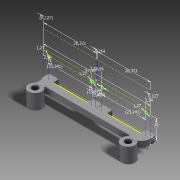
# Autodesk Inventor part: HDMIPluginModuleHolder02
Saved by Autodesk Inventor 2015 (Build 190159000, 159)
## iProperties
Created: 2015-10-14
Part Number: HDMIPluginModuleHolder02
Material: Generic
Document SubType Name: Modeling
Designer: -
Density: 1 g/cm^3
Appearance: Default
Author: -
Autodesk Inventor part; units mm, degrees
ref_plane "YZ Plane" through (0, 0, 0) normal (1, 0, 0) x (0, 1, 0)
ref_plane "XZ Plane" through (0, 0, 0) normal (0, 1, 0) x (-1, 0, 0)
ref_plane "XY Plane" through (0, 0, 0) normal (0, 0, 1) x (1, 0, 0)
sketch "Sketch1" plane through (0, 0, 0) normal (0, 1, 0) x (-1, 0, 0)
  circle A0 centre (0, 0) radius 1.65
  line L0 (0, 0) -> (22.8671, 0) construction
  circle A1 centre (-49.53, 0) radius 1.65
  circle A2 centre (-49.53, 0) radius 3.5
  line L1 (-24.765, 0) -> (-24.765, 33.4897) construction
  line L2 (0, 0) -> (0, -6.322) construction
  line L3 (-49.53, 0) -> (-44.53, 0) construction
  circle A3 centre (0, 0) radius 3.5
  dimension "d0" = 3.3
  dimension "d2" = 49.53
  dimension "d3" = 3.3
  dimension "d4" = 7
  dimension "d11" = 7
  constraints: 8 end point, 4 centre point, 3 coincident, 2 horizontal, 2 vertical, 1 point on line
  measures "d0" diameter of A0
  measures "d2" distance of L0.start A1.centre
  measures "d3" diameter of A1
  measures "d4" diameter of A2
  measures "d11" diameter of A3
extrude "Extrusion1" add sketch "Sketch1" along normal blind 3
sketch "Sketch2" plane through (49.53, 0, 0) normal (0, -1, 0) x (1, 0, 0)
  line L0 (2, -2.2) -> (2, -5.2)
  line L1 (0, -7.2) -> (-49.53, -7.2)
  line L2 (-51.53, -5.2) -> (-51.53, -2.2)
  line L3 (-47.53, -2.2) -> (-47.53, -2.2)
  line L4 (-46.53, -3.2) -> (-3, -3.2)
  line L5 (-2, -2.2) -> (-2, -2.2)
  line L6 (0, 0) -> (0, -7.7115) construction
  line L7 (2, -2.2) -> (-2, -2.2)
  line L8 (-49.53, 0) -> (-49.53, -7.2415) construction
  line L9 (-47.53, -2.2) -> (-51.53, -2.2)
  arc A0 (-47.53, -2.2) -> (-46.53, -3.2) centre (-46.53, -2.2) ccw
  arc A1 (-3, -3.2) -> (-2, -2.2) centre (-3, -2.2) ccw
  arc A2 (-51.53, -5.2) -> (-49.53, -7.2) centre (-49.53, -5.2) ccw
  arc A3 (0, -7.2) -> (2, -5.2) centre (0, -5.2) ccw
  point P0 (2, -7.2)
  point P1 (0, -2.2)
  point P2 (-49.53, -2.2)
  dimension "d14" = 5
  dimension "d15" = 2.2
  dimension "d16" = 4
  dimension "d17" = 4
  dimension "d18" = 2.2
  dimension "d19" = 1
  dimension "d20" = 2
  constraints: 20 end point, 8 point on circle, 8 tangent, 4 centre point, 4 perpendicular, 4 point on line, 3 vertical, 2 equal radius, 2 horizontal, 2 midpoint, 2 other
  measures "d14" distance of L0.start point (2, -7.2)
  measures "d15" distance from line of L6.start L7
  measures "d16" distance between parallel lines of L0 L5
  measures "d17" distance between parallel lines of L4 L1
  measures "d18" distance from line of L8.start L9
  measures "d19" radius of A0
  measures "d20" radius of A2
extrude "Extrusion2" add sketch "Sketch2" against normal blind 3.072
sketch "Sketch3" plane through (49.53, 0, -7.2) normal (0, 0, -1) x (-1, 0, 0)
  arc A0 (20.5268, 0.572) -> (21.6698, 0.572) centre (21.0983, 0.572) ccw
  line L0 (0, 0) -> (49.53, 0) construction
  line L1 (0, 3.072) -> (49.53, 3.072) projected
  line L2 (-2, 0) -> (-2, 3.072) projected
  line L3 (21.6698, 0.572) -> (21.6698, 1.207)
  line L4 (21.6698, 1.207) -> (23.6698, 1.207)
  line L5 (23.6698, 1.207) -> (23.6698, 3.072)
  line L6 (20.5268, 0.572) -> (20.5268, 1.207)
  line L7 (20.5268, 1.207) -> (18.5268, 1.207)
  line L8 (18.5268, 1.207) -> (18.5268, 3.072)
  line L9 (21.0983, 0.572) -> (22.2732, 0.572) construction
  line L10 (23.6698, 3.072) -> (18.5268, 3.072)
  point P0 (49.53, 0)
  point P1 (46.53, 3.072)
  point P2 (3, 3.072)
  dimension "d23" = 1.143
  dimension "d26" = 23.0983
  dimension "d27" = 2
  dimension "d28" = 2
  dimension "d29" = 0.635
  dimension "d30" = 0.635
  dimension "d31" = 2.5
  constraints: 16 end point, 3 perpendicular, 2 collinear, 2 horizontal, 2 point on circle, 2 point on line, 2 vertical, 1 centre point, 1 coincident, 1 tangent
  measures "d23" diameter of A0
  measures "d26" distance from line of A0.centre L2
  measures "d27" distance of L3.end L4.end
  measures "d28" distance of L6.end L7.end
  measures "d29" distance of L6.start L6.end
  measures "d30" distance of L3.start L3.end
  measures "d31" distance from line of L9.start L10
extrude "Extrusion3" add sketch "Sketch3" along normal blind 3
pattern_linear "Rectangular Pattern1" count 2 spacing 23.241 along (1, 0, 0) of "Extrusion3"
sketch "Sketch4" plane through (49.1012, 3.072, -7.2) normal (0, 1, 0) x (1, 0, 0)
  arc A0 (0, -5.143) -> (5.143, 0) centre (0, 0) ccw
  line L0 (5.143, 0) -> (0, 0)
  line L1 (0, 0) -> (0, -5.143)
  point P0 (-49.1012, -7.2)
  constraints: 4 end point, 2 point on circle, 1 centre point, 1 horizontal, 1 perpendicular
extrude "Extrusion4" add sketch "Sketch4" against normal blind 3.072
pattern_linear "Rectangular Pattern2" count 2 spacing 5.334 along (-1, 0, 0) of "Extrusion3"
pattern_linear "Rectangular Pattern3" count 2 spacing 28.575 along (-1, 0, 0) of "Extrusion3"
sketch "Sketch6" plane through (-2.7148, 3.072, -7.2) normal (0, 1, 0) x (1, 0, 0)
  arc A0 (0, 0) -> (3.143, -3.143) centre (3.143, 0) ccw
  line L0 (3.143, -3.143) -> (3.143, 0)
  line L1 (3.143, 0) -> (0, 0)
  point P0 (2.7148, -7.2)
  constraints: 4 end point, 2 point on circle, 1 centre point, 1 perpendicular, 1 vertical
extrude "Extrusion5" add sketch "Sketch6" against normal blind 3.072
sketch "Sketch7" plane through (54.2442, 3.072, -10.2) normal (0, 0, -1) x (-1, 0, 0)
  line L0 (3.143, -2.5) -> (3.143, -1.865) construction
  line L1 (3.143, -1.865) -> (5.143, -1.865) construction
  line L2 (5.143, -1.865) -> (5.143, 0) construction
  line L3 (5.143, 0) -> (0, 0) construction
  line L4 (0, 0) -> (0, -1.865) construction
  line L5 (0, -1.865) -> (2, -1.865) construction
  line L6 (2, -1.865) -> (2, -2.5) construction
  arc A0 (2, -2.5) -> (3.143, -2.5) centre (2.5715, -2.5) ccw construction
  line L7 (0, -1.865) -> (0, 0)
  line L8 (0, 0) -> (5.143, 0)
  line L9 (5.143, 0) -> (5.143, -1.865)
  arc A1 (0, -1.865) -> (5.143, -1.865) centre (2.5715, -1.865) ccw
  line L10 (5.143, -1.865) -> (0, -1.865) construction
  line L11 (5.143, -1.865) -> (5.143, 0) construction
  point P0 (54.2442, -3.072)
  constraints: 8 end point, 3 perpendicular, 2 point on circle, 1 centre point, 1 coincident, 1 midpoint, 1 vertical
extrude "Extrusion6" add sketch "Sketch7" against normal blind 1
pattern_linear "Rectangular Pattern4" count 2 spacing 23.241 along (-1, 0, 0) of "Extrusion6"
pattern_linear "Rectangular Pattern5" count 2 spacing 28.575 along (-1, 0, 0) of "Extrusion6"
pattern_linear "Rectangular Pattern6" count 2 spacing 51.816 along (-1, 0, 0) of "Extrusion6"
sketch "Sketch8" plane through (49.53, 0, -7.2) normal (0, 0, -1) x (-1, 0, 0)
  line L0 (-4.8097, 14.0243) -> (52.3403, 14.0243) construction
  line L1 (52.3403, 14.0243) -> (52.3403, 4.0243) construction
  line L2 (52.3403, 4.0243) -> (-4.8097, 4.0243) construction
  line L3 (-4.8097, 4.0243) -> (-4.8097, 14.0243) construction
  line L4 (-4.6827, 25.3025) -> (23.6383, 25.3025) construction
  line L5 (23.6383, 25.3025) -> (23.6383, 16.2547) construction
  line L6 (23.6383, 16.2547) -> (-4.6827, 16.2547) construction
  line L7 (-4.6827, 16.2547) -> (-4.6827, 25.3025) construction
  line L8 (52.2133, 25.3025) -> (23.8923, 25.3025) construction
  line L9 (23.8923, 25.3025) -> (23.8923, 16.2547) construction
  line L10 (23.8923, 16.2547) -> (52.2133, 16.2547) construction
  line L11 (52.2133, 16.2547) -> (52.2133, 25.3025) construction
  circle A0 centre (-2.1427, 14.0243) radius 0.635
  circle A1 centre (21.0983, 14.0243) radius 0.635
  circle A2 centre (26.4323, 14.0243) radius 0.635
  circle A3 centre (49.6733, 14.0243) radius 0.635
  arc A4 (-2.7142, 0.572) -> (-1.5712, 0.572) centre (-2.1427, 0.572) ccw projected
  line L12 (-2.1427, 0.572) -> (-2.1427, 10.6203) construction
  arc A5 (20.5268, 0.572) -> (21.6698, 0.572) centre (21.0983, 0.572) ccw construction
  arc A6 (25.8608, 0.572) -> (27.0038, 0.572) centre (26.4323, 0.572) ccw construction
  arc A7 (49.1018, 0.572) -> (49.53, 0.0188) centre (49.6733, 0.572) ccw construction
  line L13 (21.0983, 0.572) -> (21.0983, 9.0243) construction
  line L14 (26.4323, 0.572) -> (26.4323, 8.1687) construction
  line L15 (49.6733, 0.572) -> (49.6733, 9.0243) construction
  line L16 (23.8608, 1.207) -> (23.8608, 3.072) construction
  line L17 (23.6698, 3.072) -> (23.8608, 3.072) construction
  line L18 (23.6698, 3.072) -> (23.6698, 1.207) construction
  line L19 (23.6698, 1.207) -> (21.6698, 1.207) construction
  line L20 (21.6698, 1.207) -> (21.6698, 0.572) construction
  arc A8 (20.5268, 0.572) -> (21.6698, 0.572) centre (21.0983, 0.572) ccw construction
  line L21 (20.5268, 0.572) -> (20.5268, 1.207) construction
  line L22 (20.5268, 1.207) -> (18.5268, 1.207) construction
  line L23 (18.5268, 1.207) -> (18.5268, 3.072) construction
  line L24 (29.0038, 3.072) -> (29.0038, 1.207) construction
  line L25 (29.0038, 1.207) -> (27.0038, 1.207) construction
  line L26 (27.0038, 1.207) -> (27.0038, 0.572) construction
  arc A9 (25.8608, 0.572) -> (27.0038, 0.572) centre (26.4323, 0.572) ccw construction
  line L27 (25.8608, 0.572) -> (25.8608, 1.207) construction
  line L28 (25.8608, 1.207) -> (23.8608, 1.207) construction
  line L29 (0, 0) -> (49.53, 0) construction
  line L30 (24.765, 0) -> (24.765, 9.6631) construction
  line L31 (47.1018, 1.207) -> (47.1018, 3.072) projected
  arc A10 (49.1018, 0.572) -> (50.2448, 0.572) centre (49.6733, 0.572) ccw projected
  line L32 (49.1018, 0.572) -> (49.1018, 1.207) projected
  line L33 (49.1018, 1.207) -> (47.1018, 1.207) projected
  line L34 (0.4288, 1.207) -> (-1.5712, 1.207) projected
  line L35 (-1.5712, 1.207) -> (-1.5712, 0.572) projected
  line L36 (0.4288, 3.072) -> (18.5268, 3.072) projected
  line L37 (0.4288, 3.072) -> (0.4288, 1.207) projected
  arc A11 (-2.7142, 0.572) -> (-1.5712, 0.572) centre (-2.1427, 0.572) ccw projected
  line L38 (29.0038, 3.072) -> (47.1018, 3.072) projected
  line L39 (-2.7142, 0.572) -> (-2.7142, 1.207) projected
  line L40 (-2.7142, 1.207) -> (-4.7142, 1.207) projected
  line L41 (-4.7142, 1.207) -> (-4.7142, 0) projected
  line L42 (52.2448, 0) -> (-4.7142, 0) projected
  line L43 (52.2448, 1.207) -> (52.2448, 0) projected
  line L44 (52.2448, 1.207) -> (50.2448, 1.207) projected
  line L45 (50.2448, 1.207) -> (50.2448, 0.572) projected
  point P0 (49.53, 0)
  point P1 (49.3965, 0)
  dimension "d57" = 57.15
  dimension "d58" = 10
  dimension "d59" = 28.321
  dimension "d60" = 0.127
  dimension "d61" = 28.321
  dimension "d62" = 0.254
  dimension "d63" = 0.127
  dimension "d64" = 1.27
  dimension "d65" = 2.54
  dimension "d66" = 1.27
  dimension "d67" = 2.54
  dimension "d68" = 1.27
  dimension "d69" = 1.27
  dimension "d70" = 2.54
  dimension "d71" = 2.54
  dimension "d72" = 23.241
  dimension "d73" = 5.334
  dimension "d74" = 23.241
  dimension "d75" = 1.6673
  dimension "d76" = 3.6667
  constraints: 34 end point, 6 parallel, 5 point on line, 5 vertical, 4 centre point, 3 horizontal, 3 perpendicular, 1 collinear, 1 midpoint, 1 other
  measures "d57" distance of L0.start L0.end
  measures "d58" distance of L2.end L0.start
  measures "d59" distance of L4.start L4.end
  measures "d60" distance between parallel lines of L3 L7
  measures "d61" distance of L8.start L8.end
  measures "d62" distance between parallel lines of L5 L9
  measures "d63" distance between parallel lines of L11 L1
  measures "d64" diameter of A0
  measures "d65" distance from line of L7 A0.centre
  measures "d66" diameter of A1
  measures "d67" distance from line of A1.centre L5
  measures "d68" diameter of A3
  measures "d69" diameter of A2
  measures "d70" distance from line of L9 A2.centre
  measures "d71" distance from line of L11 A3.centre
  measures "d72" distance of A0.centre A1.centre
  measures "d73" distance of A1.centre A2.centre
  measures "d74" distance of A3.centre A2.centre
  measures "d75" distance from line of L30 A2.centre
  measures "d76" distance from line of A1.centre L30
sketch "Sketch9" plane through (0, 0, 0) normal (0, -1, 0) x (1, 0, 0)
  circle A0 centre (0, 0) radius 1.65 projected
  circle A1 centre (49.53, 0) radius 1.65 projected
  circle A2 centre (49.53, 0) radius 3.5
  arc A3 (2.1649, -2.7501) -> (-2, -2.8723) centre (0, 0) ccw projected
  circle A4 centre (0, 0) radius 3.5
  constraints: 2 centre point, 2 coincident
extrude "Extrusion7" add sketch "Sketch9" along normal blind 5
body "Solid1"
